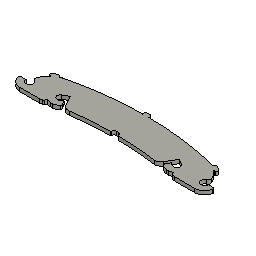
top-piece (Autodesk Fusion 360 design; units mm, degrees)
Autodesk Fusion 360 part; units mm, degrees
note: some values were not read from the file. Set by a fixed rule: which sketch regions a step uses.
(part 1 of 2)
sketch "Main body" plane through (0, 0, 0) normal (0, 0, 1) x (1, 0, 0)
  line L0 (0, 0) -> (0, 30.7494) construction
  line L1 (60, 23.4426) -> (-60, 23.4426) construction
  line L2 (-70, 13.4426) -> (70, 13.4426) construction
  line L3 (-70, 13.4426) -> (-70, 0) construction
  line L4 (70, 0) -> (70, 13.4426) construction
  line L5 (-77.5, 7.9426) -> (77.5, 7.9426) construction
  circle A0 centre (-70, 7.9426) radius 2.9426 construction
  arc A1 (-77.8598, 6.7985) -> (-70, 0) centre (-70, 7.9426) ccw
  line L6 (-76.8702, 7.9426) -> (-72.9426, 7.9426)
  arc A2 (-76.8702, 7.9426) -> (-77.8598, 6.7985) centre (-76.8702, 6.9426) ccw
  circle A3 centre (70, 7.9426) radius 2.9426 construction
  line L7 (72.9426, 7.9426) -> (76.8702, 7.9426)
  arc A4 (70, 0) -> (77.8598, 6.7985) centre (70, 7.9426) ccw
  arc A5 (77.8598, 6.7985) -> (76.8702, 7.9426) centre (76.8702, 6.9426) ccw
  arc A6 (-72.9426, 7.9426) -> (-68.8487, 10.6506) centre (-70, 7.9426) ccw
  arc A7 (68.8487, 10.6506) -> (72.9426, 7.9426) centre (70, 7.9426) ccw
  line L8 (-77.5, 30.7494) -> (77.5, 30.7494) construction
  line L9 (77.5, 30.7494) -> (77.5, 0) construction
  line L10 (77.5, 0) -> (-77.5, 0) construction
  line L11 (-77.5, 0) -> (-77.5, 30.7494) construction
  line L12 (-60, 23.4426) -> (-60, 13.4426) construction
  line L13 (60, 23.4426) -> (60, 13.4426) construction
  line L14 (-70, 0) -> (70, 0)
  arc A8 (59.6571, 23.5271) -> (-59.6571, 23.5271) centre (0, -219.2506) ccw
  arc A9 (-60.3719, 23.2864) -> (-70, 13.4426) centre (-53.134, 6.5765) ccw
  arc A10 (-70, 13.4426) -> (-68.8487, 10.6506) centre (-68.0067, 12.6311) ccw
  line L15 (-60, 13.4426) -> (-66.0104, 19.453) construction
  arc A11 (70, 13.4426) -> (60.3719, 23.2864) centre (53.134, 6.5765) ccw
  line L16 (66.0105, 19.4529) -> (60, 13.4426) construction
  arc A12 (68.8487, 10.6506) -> (70, 13.4426) centre (68.0067, 12.6311) ccw
  arc A13 (-59.6571, 23.5271) -> (-60.3719, 23.2864) centre (-58.5833, 19.1571) ccw
  arc A14 (60.3719, 23.2864) -> (59.6571, 23.5271) centre (58.5833, 19.1571) ccw
  point P0 (0, 13.4426)
  point P1 (0, 7.9426)
  point P2 (70, 7.9426)
  point P3 (-72.9426, 7.9426)
  point P4 (72.9426, 7.9426)
  point P5 (-77.5, 7.9426)
  point P6 (-77.5, 13.4426)
  point P7 (-77.5, 23.4426)
  point P8 (-70, 0)
  point P9 (0, 30.7494)
  point P10 (-70, 30.7494)
  point P11 (-60, 30.7494)
  point P12 (0, 30.2837)
  point P13 (-66.6872, 16.948)
  point P14 (-66.0104, 19.453)
  dimension "d450" = 5.8852
  dimension "d456" = 1
  dimension "d457" = 5.8852
  dimension "d458" = 1
  dimension "d459" = 7.9426
  dimension "d460" = 5.5
  dimension "d461" = 10
  dimension "d463" = 70
  dimension "d465" = 7.5
  dimension "d467" = 10
  dimension "d520" = 250
  dimension "d551" = 8.5
  dimension "d552" = 8.5
  dimension "d561" = 4.5
  dimension "d562" = 4.5
  dimension "d572" = 2.1521
  dimension "d573" = 2.1521
  dimension "d574" = 10
  constraint coincident L0.start origin
  constraint vertical L0
  constraint perpendicular L0 L1
  constraint horizontal L2
  constraint coincident L2 P0
  constraint midpoint L2 P0
  constraint coincident L0 P0
  constraint perpendicular L2 L3
  constraint perpendicular L4 L5
  constraint coincident L5 P1
  constraint midpoint L5 P1
  constraint coincident L0 P1
  constraint coincident L5 A0.centre
  constraint coincident L3 A0.centre
  constraint coincident L5 P2
  constraint coincident L4 P2
  constraint coincident A0.centre A1.centre
  constraint coincident L5 L6.start
  constraint coincident L5 P3
  constraint parallel L5 L6
  constraint coincident A0 P3
  constraint coincident P3 L6.end
  constraint coincident A1.start A2.end
  constraint tangent L6 A2
  constraint tangent A1 A2
  constraint coincident P2 A3.centre
  constraint coincident L5 P4
  constraint coincident L5 L7.end
  constraint parallel L5 L7
  constraint coincident A3 P4
  constraint coincident P4 L7.start
  constraint tangent L5 A5
  constraint tangent A4 A5
  constraint coincident A0 A6.end
  constraint horizontal L8
  constraint vertical L9
  constraint horizontal L10
  constraint vertical L11
  constraint coincident L11 P5
  constraint coincident L11 P6
  constraint coincident L11 P7
  constraint coincident L10 P8
  constraint midpoint L0.start L10
  constraint coincident L5 P5
  constraint coincident L2 P6
  constraint coincident L1 P7
  constraint midpoint L8 P9
  constraint coincident L8 P10
  constraint coincident L3 P10
  constraint coincident P5 L5.start
  constraint coincident L3 P8
  constraint coincident P9 L0.end
  constraint coincident L2 L12.end
  constraint perpendicular L2 L12
  constraint coincident L2 L13.end
  constraint perpendicular L2 L13
  constraint coincident L8 P11
  constraint coincident L12 P11
  constraint coincident A1 P8
  constraint coincident L4.start L10
  constraint coincident P8 L3.end
  constraint perpendicular L0 L5
  constraint coincident L0 P12
  constraint tangent A9 A10
  constraint tangent A0 A10
  constraint coincident P14 L15.end
  constraint tangent A11 A12
  constraint tangent A7 A12
  constraint coincident P9 A8
  constraint coincident A9 P14
  constraint coincident L1.end A8
  constraint coincident L1.end A9
  constraint tangent A8 A13
  constraint tangent A9 A13
  constraint coincident A11 L16.start
  constraint coincident L1.start A8
  constraint coincident L1.start A11
  constraint tangent A8 A14
  constraint tangent A11 A14
  measures "d450" diameter of A0
  measures "d456" radius of A2
  measures "d457" diameter of A3
  measures "d458" radius of A5
  measures "d459" distance of L10.end P5
  measures "d460" distance of P5 P6
  measures "d461" distance of P6 P7
  measures "d463" distance of P9 P10
  measures "d465" distance of L8.start P10
  measures "d467" distance of P10 P11
  measures "d520" radius of A8
  measures "d551" distance of L12.end P14
  measures "d552" distance of L13.end L16.start
  measures "d561" radius of A13
  measures "d562" radius of A14
  measures "d572" radius of A12
  measures "d573" radius of A10
  measures "d574" distance of L2.end L13.end
sketch "Inner connectors _ old" plane through (0, 0, 0) normal (0, 0, 1) x (1, 0, 0)
  line L0 (-77.5, 7.9426) -> (77.5, 7.9426) construction
  line L1 (77.5, 0) -> (-77.5, 0) construction
  line L2 (-77.5, 0) -> (77.5, 0) construction
  line L3 (-35.4314, 0) -> (-43.4022, 13.8057)
  line L4 (-37.9718, 0) -> (-42.5574, 7.9426) construction
  line L5 (-43.5574, 7.9426) -> (-42.5574, 7.9426) construction
  line L6 (-40.6522, 9.0426) -> (-42.5574, 7.9426) construction
  arc A0 (-45.5, 5.1751) -> (-43.5574, 7.9426) centre (-46.5, 7.9426) ccw
  arc A1 (-46.5, 0) -> (-40.3845, 2.8745) centre (-46.5, 7.9426) ccw
  line L7 (-46.5, 7.9426) -> (-46.5, 0) construction
  arc A2 (-40.3845, 2.8745) -> (-40.2884, 4.0126) centre (-41.1545, 3.5126) ccw
  line L8 (-46.5, 0) -> (-35.4314, 0)
  line L9 (35.6624, 0) -> (43.5754, 13.7057)
  line L10 (37.9718, 0) -> (42.5574, 7.9426) construction
  line L11 (43.5574, 7.9426) -> (42.5574, 7.9426) construction
  line L12 (42.5574, 7.9426) -> (40.8254, 8.9426) construction
  arc A3 (43.5574, 7.9426) -> (45.5, 5.1751) centre (46.5, 7.9426) ccw
  arc A4 (40.3845, 2.8745) -> (46.5, 0) centre (46.5, 7.9426) ccw
  arc A5 (40.2884, 4.0126) -> (40.3845, 2.8745) centre (41.1545, 3.5126) ccw
  line L13 (46.5, 7.9426) -> (46.5, 0) construction
  line L14 (35.6624, 0) -> (46.5, 0)
  line L15 (-47.5, 5.1751) -> (-45.5, 5.1751)
  line L16 (-40.2884, 4.0126) -> (-42.0574, 7.0766)
  arc A6 (-42.0574, 7.0766) -> (-43.5574, 7.9426) centre (-43.5574, 6.2105) ccw
  line L17 (40.2884, 4.0126) -> (42.0574, 7.0766)
  arc A7 (43.5574, 7.9426) -> (42.0574, 7.0766) centre (43.5574, 6.2105) ccw
  line L18 (47.5, 5.1751) -> (45.5, 5.1751)
  line L19 (43.5754, 13.7057) -> (47.3852, 11.5061)
  arc A8 (-49.4426, 7.9426) -> (-47.5, 5.1751) centre (-46.5, 7.9426) ccw
  line L20 (-43.4022, 13.8057) -> (-47.3852, 11.5061)
  arc A9 (-47.3852, 11.5061) -> (-49.4426, 7.9426) centre (-45.3277, 7.9426) ccw
  arc A10 (47.5, 5.1751) -> (49.4426, 7.9426) centre (46.5, 7.9426) ccw
  arc A11 (49.4426, 7.9426) -> (47.3852, 11.5061) centre (45.3277, 7.9426) ccw
  point P0 (-70, 7.9426)
  point P1 (70, 7.9426)
  point P2 (-46.5, 5.1751)
  point P3 (46.5, 5.1751)
  point P4 (-43.4022, 13.8057)
  dimension "d469" = 23.5
  dimension "d471" = 23.5
  dimension "d486" = 60
  dimension "d487" = 2.2
  dimension "d488" = 1
  dimension "d492" = 1
  dimension "d493" = 60
  dimension "d495" = 1
  dimension "d498" = 2
  dimension "d500" = 1
  dimension "d571" = 5
  dimension "d575" = 2.9426
  dimension "d577" = 1
  dimension "d578" = 1
  dimension "d579" = 2.9426
  dimension "d585" = 5
  constraint coincident L1.end L2.start
  constraint coincident L1.start L2.end
  constraint coincident L1 L3.start
  constraint coincident L1 L4.start
  constraint parallel L3 L4
  constraint coincident L0 L5.start
  constraint parallel L0 L5
  constraint coincident L3 L6.start
  constraint perpendicular L3 L6
  constraint coincident L2 A1.start
  constraint coincident A0.centre A1.centre
  constraint vertical L7
  constraint tangent A1 A2
  constraint coincident L4 A2.end
  constraint coincident L2 L9.start
  constraint coincident L2 L10.start
  constraint parallel L9 L10
  constraint coincident L0 L11.start
  constraint parallel L0 L11
  constraint perpendicular L10 L12
  constraint coincident L9 L12.end
  constraint coincident L2 A4.end
  constraint coincident A3.centre A4.centre
  constraint coincident L10 A5.start
  constraint tangent L10 A5
  constraint tangent A4 A5
  constraint coincident L1 A4.end
  constraint perpendicular L1 L13
  constraint coincident A0 L15.end
  constraint horizontal L15
  constraint coincident L4 L16.end
  constraint tangent A2 L16
  constraint parallel L4 L16
  constraint tangent L16 A6
  constraint coincident L10 L17.end
  constraint parallel L10 L17
  constraint tangent L17 A7
  constraint tangent L0 A6
  constraint tangent L0 A7
  constraint coincident A3 L18.end
  constraint horizontal L18
  constraint perpendicular L9 L19
  constraint coincident A0.start L15.end
  constraint coincident L0 A0.centre
  constraint midpoint L15 P2
  constraint coincident L7 P2
  constraint coincident L0 A3.centre
  constraint midpoint L18 P3
  constraint coincident L13 P3
  constraint coincident A3.end L18.end
  constraint coincident P4 L3.end
  constraint coincident L0 A8.start
  constraint coincident A8.start A9.end
  constraint coincident L20.end A9.start
  constraint tangent A8 A9
  constraint tangent L20 A9
  constraint perpendicular L3 L20
  constraint tangent A10 A11
  constraint tangent L19 A11
  constraint coincident L0 A10.end
  measures "d469" distance of P0 A0.centre
  measures "d471" distance of P1 A3.centre
  measures "d486" angle of L2 L3
  measures "d487" distance of L3 L4
  measures "d488" distance of L5.start L4.end
  measures "d492" radius of A2
  measures "d493" angle of L2 L10
  measures "d495" distance of L11.start L10.end
  measures "d498" distance of L10.end L12.end
  measures "d500" radius of A5
  measures "d571" distance of L11.start L19
  measures "d575" radius of A0
  measures "d577" distance of L15.start P2
  measures "d578" distance of L13 A3.end
  measures "d579" radius of A3
  measures "d585" distance of L5.start L20
sketch "Inner curve" plane through (0, 0, 0) normal (0, 0, 1) x (1, 0, 0)
  line L0 (-70, 0) -> (70, 0) construction
  line L1 (0, 30.7494) -> (0, 0) construction
  arc A0 (59.6571, 23.5271) -> (-59.6571, 23.5271) centre (0, -219.2506) ccw
  arc A1 (53.3069, 0) -> (-53.3069, 0) centre (0, -244.2506) ccw
  line L2 (-70, 0) -> (70, 0) construction
  line L3 (-53.3069, 0) -> (53.3069, 0)
  point P0 (0, 30.7494)
  point P1 (0, 5.7494)
  dimension "d505" = 25
  dimension "d586" = 250
  constraint coincident P0 L1.start
  constraint coincident L1.end origin
  constraint coincident L1 P1
  constraint coincident L0 A1.start
  constraint coincident L0 A1.end
  constraint midpoint P1 A1
  constraint coincident L0.start L2.start
  constraint coincident L0.end L2.end
  measures "d505" distance of P0 P1
  measures "d586" radius of A1
sketch "Spike top" plane through (0, 0, 0) normal (0, 0, 1) x (1, 0, 0)
  arc A0 (-1, 33.2494) -> (-2.5, 31.7494) centre (-1, 31.7494) ccw
  line L0 (2.5, 31.7494) -> (2.5, 30.7369)
  line L1 (-1, 33.2494) -> (1, 33.2494)
  arc A1 (2.5, 31.7494) -> (1, 33.2494) centre (1, 31.7494) ccw
  line L2 (-2.5, 30.7369) -> (-2.5, 31.7494)
  line L3 (0, 0) -> (0, 33.2494) construction
  arc A2 (59.6571, 23.5271) -> (-59.6571, 23.5271) centre (0, -219.2506) ccw
  point P0 (2.5, 33.2494)
  point P1 (-2.5, 33.2494)
  point P2 (0, 30.7494)
  dimension "d196" = 5
  dimension "d198" = 1.5
  dimension "d199" = 1.5
  dimension "d522" = 2.5
  constraint vertical L2
  constraint perpendicular L1 L2
  constraint vertical L0
  constraint coincident P1 L2
  constraint coincident P1 L1
  constraint tangent A0 L2
  constraint tangent A0 L1
  constraint coincident P0 L1
  constraint coincident P0 L0
  constraint tangent L1 A1
  constraint tangent L0 A1
  constraint coincident L3.start origin
  constraint vertical L3
  constraint midpoint L1 L3.end
  constraint coincident L2.start A2
  constraint coincident L0.end A2
  constraint coincident P2 A2
  measures "d196" distance of P0 P1
  measures "d198" radius of A0
  measures "d199" radius of A1
  measures "d522" distance of L3.end P2
sketch "Spike side" plane through (0, 0, 0) normal (0, 0, 1) x (1, 0, 0)
  line L0 (-64.6665, 23.7784) -> (-63.2744, 21.7019) construction
  line L1 (-66.8617, 22.3068) -> (-62.4714, 25.2501) construction
  line L2 (-66.8617, 22.3068) -> (-68.0588, 21.5042) construction
  line L3 (-62.4714, 25.2501) -> (-61.2782, 22.8639) construction
  line L4 (-68.0588, 21.5042) -> (-66.0092, 19.4542) construction
  arc A0 (-61.4625, 23.2324) -> (-64.3452, 23.9939) centre (-63.2391, 22.344) ccw
  arc A1 (-66.5432, 22.5203) -> (-66.7687, 20.2138) centre (-65.7079, 21.2744) ccw
  line L5 (-66.5432, 22.5203) -> (-64.3452, 23.9939)
  line L6 (-61.4625, 23.2324) -> (-61.2782, 22.8639)
  line L7 (-66.4461, 19.8912) -> (-61.4625, 23.2324) construction
  line L8 (-65.6155, 20.4481) -> (-65.3622, 20.0701)
  line L9 (-65.6155, 20.4481) -> (-66.4461, 19.8912)
  line L10 (-66.7687, 20.2138) -> (-66.4461, 19.8912)
  line L11 (66.8617, 22.3068) -> (62.4714, 25.2501) construction
  line L12 (66.4461, 19.8912) -> (61.4625, 23.2324) construction
  line L13 (66.8617, 22.3068) -> (68.0588, 21.5042) construction
  line L14 (64.6665, 23.7784) -> (63.2744, 21.7019) construction
  line L15 (62.4714, 25.2501) -> (61.2782, 22.8639) construction
  line L16 (65.6155, 20.4481) -> (66.4461, 19.8912)
  arc A2 (66.5432, 22.5203) -> (66.7687, 20.2138) centre (65.7079, 21.2744) cw
  line L17 (66.5432, 22.5203) -> (64.3452, 23.9939)
  line L18 (65.6155, 20.4481) -> (65.3622, 20.0701)
  arc A3 (61.4625, 23.2324) -> (64.3452, 23.9939) centre (63.2391, 22.344) cw
  line L19 (61.4625, 23.2324) -> (61.2782, 22.8639)
  line L20 (68.0588, 21.5042) -> (66.0092, 19.4542) construction
  line L21 (66.7687, 20.2138) -> (66.4461, 19.8912)
  arc A4 (-60.3719, 23.2864) -> (-70, 13.4426) centre (-53.134, 6.5765) ccw
  arc A5 (70, 13.4426) -> (60.3719, 23.2864) centre (53.134, 6.5765) ccw
  point P0 (0, 47.6931)
  point P1 (0, 45.6174)
  point P2 (-53.134, 6.5765)
  point P3 (-66.0104, 19.453)
  point P4 (53.134, 6.5765)
  point P5 (66.0105, 19.4529)
  dimension "d314" = 2.5
  dimension "d321" = 1.5
  dimension "d323" = 2.5
  dimension "d327" = 1.5
  dimension "d553" = 0.455
  dimension "d554" = 0.455
  dimension "d555" = 5
  dimension "d556" = 1
  dimension "d557" = 5
  dimension "d558" = 1
  dimension "d559" = 1
  dimension "d560" = 1
  constraint midpoint L0.start L1
  constraint perpendicular L0 L1
  constraint collinear L1 L2
  constraint tangent L1 A0
  constraint coincident L3 A0.start
  constraint coincident L1 A0.end
  constraint tangent L3 A0
  constraint coincident L4 A1.end
  constraint coincident L1 A1.start
  constraint tangent L1 A1
  constraint tangent L4 A1
  constraint coincident L4 L7.start
  constraint coincident L7 L8.start
  constraint perpendicular L7 L8
  constraint coincident L1.start L8
  constraint midpoint L14.start L11
  constraint perpendicular L11 L14
  constraint collinear L11 L13
  constraint tangent L11 A3
  constraint coincident L12.end L15
  constraint coincident L17.end L11
  constraint tangent L15 A3
  constraint coincident A2.end L20
  constraint coincident A2.start L11
  constraint tangent L11 A2
  constraint tangent A2 L20
  constraint coincident L12.start L20
  constraint coincident L16.start L12
  constraint perpendicular L12 L18
  constraint coincident L11.start L18
  constraint perpendicular L0 L7
  constraint coincident L12.end L19
  constraint perpendicular L12 L14
  constraint coincident L3.end A4
  constraint coincident L0.end A4
  constraint coincident L4.end A4
  constraint coincident L0 P2
  constraint coincident L14 P4
  constraint coincident L18.end A5
  constraint coincident L20.end A5
  constraint coincident L14.end A5
  constraint coincident L15 P4
  constraint coincident L20 P4
  constraint coincident L4 P2
  constraint coincident L3 P2
  constraint coincident L8.end A4
  constraint coincident A5 L15.end
  measures "d314" distance of L0.start L0.end
  measures "d321" radius of A1
  measures "d323" distance of L14.end L14.start
  measures "d327" radius of A2
  measures "d553" distance of L8.start L8.end
  measures "d554" distance of L18.end L16.start
  measures "d555" distance of A0.start L8.start
  measures "d556" distance of L7.start L8.start
  measures "d557" distance of L12.end L16.start
  measures "d558" distance of L12.start L16.start
  measures "d559" distance of L3.end A4.start
  measures "d560" distance of A5.end L15.end
sketch "Inner connector" plane through (0, 0, 0) normal (0, 0, 1) x (1, 0, 0)
  arc A0 (53.3069, 0) -> (-53.3069, 0) centre (0, -244.2506) ccw
  line L0 (-70, 7.9426) -> (-46.5, 7.9426) construction
  line L1 (-46.5, 9.4539) -> (-46.5, 1.3868) construction
  arc A1 (-45.5, 6.6865) -> (-43.9516, 7.9827) centre (-46.5, 9.4539) ccw
  line L2 (-45.5, 6.6865) -> (-47.5, 6.6865)
  arc A2 (-49.0248, 7.9426) -> (-47.5, 6.6865) centre (-46.5, 9.4539) ccw
  line L3 (-39.0403, 5.876) -> (-43.6804, 13.9128)
  line L4 (-46.5, 9.4539) -> (-51.7672, 0.331) construction
  line L5 (-43.6804, 13.9128) -> (-48.1443, 11.3355)
  line L6 (-46.5, 9.4539) -> (-43.9516, 7.9827) construction
  line L7 (-43.9516, 7.9827) -> (-43.0856, 8.4827)
  line L8 (-45.5, 6.6865) -> (-45.5, 1.6865) construction
  line L9 (-47.5, 6.6865) -> (-47.5, 1.6865) construction
  line L10 (-47.5, 1.6865) -> (-45.5, 1.6865)
  arc A3 (-45.5, 1.6865) -> (-41.2154, 3.6741) centre (-46.5, 9.4539) ccw
  arc A4 (-50.4158, 2.6716) -> (-47.5, 1.6865) centre (-46.5, 9.4539) ccw
  line L11 (-50.4158, 2.6716) -> (-51.4694, 0.8467)
  arc A5 (-48.1443, 11.3355) -> (-49.0248, 7.9426) centre (-46.9147, 9.2057) ccw
  line L12 (-43.0856, 8.4827) -> (-41.0242, 4.9121)
  arc A6 (-41.2154, 3.6741) -> (-41.0242, 4.9121) centre (-41.8902, 4.4121) ccw
  arc A7 (-39.0403, 5.876) -> (-34.0296, 3.4225) centre (-34.7102, 8.376) ccw
  line L13 (0, 0) -> (0, 5.7494)
  arc A8 (47.5, 1.6865) -> (50.4158, 2.6716) centre (46.5, 9.4539) ccw
  line L14 (47.5, 1.6865) -> (45.5, 1.6865)
  arc A9 (41.2154, 3.6741) -> (45.5, 1.6865) centre (46.5, 9.4539) ccw
  arc A10 (41.0242, 4.9121) -> (41.2154, 3.6741) centre (41.8902, 4.4121) ccw
  line L15 (43.0856, 8.4827) -> (41.0242, 4.9121)
  line L16 (43.9516, 7.9827) -> (43.0856, 8.4827)
  arc A11 (43.9516, 7.9827) -> (45.5, 6.6865) centre (46.5, 9.4539) ccw
  line L17 (45.5, 6.6865) -> (47.5, 6.6865)
  arc A12 (47.5, 6.6865) -> (49.0248, 7.9426) centre (46.5, 9.4539) ccw
  arc A13 (49.0248, 7.9426) -> (48.1443, 11.3355) centre (46.9147, 9.2057) ccw
  line L18 (43.6804, 13.9128) -> (48.1443, 11.3355)
  line L19 (39.0403, 5.876) -> (43.6804, 13.9128)
  arc A14 (34.0296, 3.4225) -> (39.0403, 5.876) centre (34.7102, 8.376) ccw
  line L20 (-45.5, 1.6865) -> (-45.5, 1.574) construction
  line L21 (77.5, 0) -> (-77.5, 0) construction
  line L22 (-51.7672, 0.331) -> (-53.3069, 0) construction
  arc A15 (-52.1253, 0.3691) -> (-51.4694, 0.8467) centre (-52.3354, 1.3467) ccw
  line L23 (-53.8422, 0) -> (-52.1253, 0.3691)
  line L24 (-53.3069, 0) -> (-53.8422, 0)
  line L25 (50.4158, 2.6716) -> (51.4694, 0.8467)
  arc A16 (51.4694, 0.8467) -> (52.1253, 0.3691) centre (52.3354, 1.3467) ccw
  line L26 (53.8422, 0) -> (52.1253, 0.3691)
  line L27 (53.3069, 0) -> (53.8422, 0)
  point P0 (-70, 7.9426)
  point P1 (-46.5, 6.6865)
  point P2 (-45.5, 6.6865)
  dimension "d598" = 23.5
  dimension "d617" = 2.9426
  dimension "d618" = 2
  dimension "d620" = 1
  dimension "d623" = 30
  dimension "d624" = 5
  dimension "d625" = 60
  dimension "d633" = 30
  dimension "d634" = 2.2
  dimension "d635" = 1
  dimension "d637" = 5
  dimension "d639" = 23.5
  dimension "d658" = 0.1125
  dimension "d662" = 1
  dimension "d663" = 5
  dimension "d664" = 0.1125
  constraint coincident P0 L0.start
  constraint coincident L0.end L1
  constraint coincident A0 L1.end
  constraint vertical L1
  constraint horizontal L0
  constraint coincident L1 A1.centre
  constraint perpendicular L1 L2
  constraint midpoint L2 P1
  constraint coincident L1 P1
  constraint coincident P2 A1.start
  constraint coincident L1.start A1.centre
  constraint coincident A0 L4.end
  constraint perpendicular L3 L5
  constraint perpendicular L2 L8
  constraint perpendicular L2 L9
  constraint horizontal L10
  constraint parallel L4 L11
  constraint tangent L5 A5
  constraint tangent A2 A5
  constraint coincident L0 A2.start
  constraint perpendicular L7 L12
  constraint parallel L3 L12
  constraint tangent L12 A6
  constraint tangent A3 A6
  constraint tangent L3 A7
  constraint coincident A0 A7.end
  constraint tangent A0 A7
  constraint coincident L13.start origin
  constraint midpoint A0 L13.end
  constraint symmetric P2 L13 A11.end
  constraint symmetric A1.end L13 L16.start
  constraint symmetric A1 L13 A11
  constraint symmetric L2.end L13 L17.end
  constraint symmetric A2.start L13 A12.end
  constraint symmetric A2 L13 A12
  constraint symmetric L3.start L13 L19.start
  constraint symmetric L3.end L13 L18.start
  constraint symmetric L5.end L13 A13.end
  constraint symmetric L7.end L13 L15.start
  constraint symmetric L8.end L13 L14.end
  constraint symmetric L9.end L13 A8.start
  constraint symmetric A3.end L13 A9.start
  constraint symmetric A3 L13 A9
  constraint symmetric A4.start L13 A8.end
  constraint symmetric A4 L13 A8
  constraint symmetric A5 L13 A13
  constraint symmetric L12.end L13 A10.start
  constraint symmetric A6 L13 A10
  constraint symmetric A7.end L13 A14.start
  constraint symmetric A7 L13 A14
  constraint coincident A0 L20.end
  constraint perpendicular L10 L20
  constraint coincident L8.end L10.end
  constraint coincident A0.end L22.end
  constraint coincident L21 L23.start
  constraint tangent L4 A15
  constraint coincident L4 L11.end
  constraint coincident L11 A15.end
  constraint parallel L22 L23
  constraint parallel L21 L24
  constraint coincident L11.end A15.end
  constraint tangent A15 L23
  constraint symmetric L13 A0.end A0.start
  constraint symmetric L13 L23.start L26.start
  constraint symmetric L13 L11.end L25.end
  constraint symmetric L13 A15.start A16.end
  constraint symmetric L13 A15 A16
  measures "d598" distance of P0 L0.end
  measures "d617" radius of A1
  measures "d618" distance of P2 L2.end
  measures "d620" distance of A1.end L7.end
  measures "d623" angle of L1 L4
  measures "d624" distance of A1.end L5
  measures "d625" angle of L1 L6
  measures "d633" angle of L1 L3
  measures "d634" distance of L3 L7.end
  measures "d635" radius of A6
  measures "d637" radius of A7
  measures "d639" distance of P0 L0.end
  measures "d658" distance of L8.end L20.end
  measures "d662" radius of A15
  measures "d663" distance of P2 L8.end
  measures "d664" distance of L22 L23
extrude "Extrude6" add sketch "Spike top" sketch "Main body" sketch "Spike side" along normal blind 3 of sketch 2 of sketch 3 makes body 1
extrude "Extrude7" cut sketch "Inner connector" sketch "Inner curve" along normal blind 3 of sketch 2 bodies 1
copy_body "CopyPasteBodies6" bodies 1 makes body 2
move_body "Move9" bodies 2 to x (1, 0, 0) y (0, 1, 0) z (0, 0, 1) at (0, -25.45, 0)
sketch "Cutouts" plane through (0, 0, 0) normal (0, 0, 1) x (1, 0, 0)
  line L0 (-70, 0) -> (70, 0)
  arc A0 (-1, 7.7994) -> (-2.5, 6.2994) centre (-1, 6.2994) ccw construction
  line L1 (-2.5, 6.2994) -> (-2.5, 5.2869) construction
  line L2 (1, 7.7994) -> (-1, 7.7994) construction
  arc A1 (2.5, 6.2994) -> (1, 7.7994) centre (1, 6.2994) ccw construction
  line L3 (2.5, 5.2869) -> (2.5, 6.2994) construction
  line L4 (2.95, 5.2869) -> (2.95, 6.2994)
  arc A2 (2.95, 6.2994) -> (1, 8.2494) centre (1, 6.2994) ccw
  line L5 (1, 8.2494) -> (-1, 8.2494)
  arc A3 (-1, 8.2494) -> (-2.95, 6.2994) centre (-1, 6.2994) ccw
  line L6 (-2.95, 6.2994) -> (-2.95, 5.2869)
  line L7 (-2.95, 5.2869) -> (-2.95, 0)
  line L8 (2.95, 5.2869) -> (2.95, 0)
  dimension "d527" = 0.45
  constraint coincident L0 L7.end
  constraint perpendicular L0 L7
  constraint coincident L0 L8.end
  constraint perpendicular L0 L8
extrude "Extrude8" cut sketch "Cutouts" along normal blind 3 bodies 1
delete_body "RemoveBody3" bodies 2
sketch "Without inner connectors" plane through (0, 0, 0) normal (0, 0, 1) x (1, 0, 0)
  line L0 (2.95, 6.2994) -> (2.95, 5.732)
  line L1 (53.3069, 0) -> (70, 0)
  arc A0 (70, 0) -> (77.8598, 6.7985) centre (70, 7.9426) ccw
  arc A1 (77.8598, 6.7985) -> (76.8702, 7.9426) centre (76.8702, 6.9426) ccw
  line L2 (76.8702, 7.9426) -> (72.9426, 7.9426)
  arc A2 (68.8487, 10.6506) -> (72.9426, 7.9426) centre (70, 7.9426) ccw
  arc A3 (68.8487, 10.6506) -> (70, 13.4426) centre (68.0067, 12.6311) ccw
  arc A4 (70, 13.4426) -> (65.3622, 20.0701) centre (53.134, 6.5765) ccw
  line L3 (65.3622, 20.0701) -> (65.6155, 20.4481)
  line L4 (65.6155, 20.4481) -> (66.4461, 19.8912)
  line L5 (66.4461, 19.8912) -> (66.7687, 20.2138)
  arc A5 (66.7687, 20.2138) -> (66.5432, 22.5203) centre (65.7079, 21.2744) ccw
  line L6 (66.5432, 22.5203) -> (64.3452, 23.9939)
  arc A6 (64.3452, 23.9939) -> (61.4625, 23.2324) centre (63.2391, 22.344) ccw
  line L7 (61.4625, 23.2324) -> (61.2782, 22.8639)
  arc A7 (61.2782, 22.8639) -> (60.3719, 23.2864) centre (53.134, 6.5765) ccw
  arc A8 (60.3719, 23.2864) -> (59.6571, 23.5271) centre (58.5833, 19.1571) ccw
  arc A9 (59.6571, 23.5271) -> (2.5, 30.7369) centre (0, -219.2506) ccw
  line L8 (2.5, 30.7369) -> (2.5, 31.7494)
  arc A10 (2.5, 31.7494) -> (1, 33.2494) centre (1, 31.7494) ccw
  line L9 (1, 33.2494) -> (-1, 33.2494)
  arc A11 (-1, 33.2494) -> (-2.5, 31.7494) centre (-1, 31.7494) ccw
  line L10 (-2.5, 31.7494) -> (-2.5, 30.7369)
  arc A12 (-2.5, 30.7369) -> (-59.6571, 23.5271) centre (0, -219.2506) ccw
  arc A13 (-59.6571, 23.5271) -> (-60.3719, 23.2864) centre (-58.5833, 19.1571) ccw
  arc A14 (-60.3719, 23.2864) -> (-61.2782, 22.8639) centre (-53.134, 6.5765) ccw
  line L11 (-61.2782, 22.8639) -> (-61.4625, 23.2324)
  arc A15 (-61.4625, 23.2324) -> (-64.3452, 23.9939) centre (-63.2391, 22.344) ccw
  line L12 (-64.3452, 23.9939) -> (-66.5432, 22.5203)
  arc A16 (-66.5432, 22.5203) -> (-66.7687, 20.2138) centre (-65.7079, 21.2744) ccw
  line L13 (-66.7687, 20.2138) -> (-66.4461, 19.8912)
  line L14 (-66.4461, 19.8912) -> (-65.6155, 20.4481)
  line L15 (-65.6155, 20.4481) -> (-65.3622, 20.0701)
  arc A17 (-65.3622, 20.0701) -> (-70, 13.4426) centre (-53.134, 6.5765) ccw
  arc A18 (-70, 13.4426) -> (-68.8487, 10.6506) centre (-68.0067, 12.6311) ccw
  arc A19 (-72.9426, 7.9426) -> (-68.8487, 10.6506) centre (-70, 7.9426) ccw
  line L16 (-72.9426, 7.9426) -> (-76.8702, 7.9426)
  arc A20 (-76.8702, 7.9426) -> (-77.8598, 6.7985) centre (-76.8702, 6.9426) ccw
  arc A21 (-77.8598, 6.7985) -> (-70, 0) centre (-70, 7.9426) ccw
  line L17 (-70, 0) -> (-53.3069, 0)
  line L18 (-2.95, 5.732) -> (-2.95, 6.2994)
  arc A22 (-1, 8.2494) -> (-2.95, 6.2994) centre (-1, 6.2994) ccw
  line L19 (-1, 8.2494) -> (1, 8.2494)
  arc A23 (2.95, 6.2994) -> (1, 8.2494) centre (1, 6.2994) ccw
  arc A24 (41.3805, 2.3009) -> (36.4767, 3.0739) centre (0, -244.2506) ccw
  arc A25 (-36.4767, 3.0739) -> (-41.0722, 2.3524) centre (0, -244.2506) ccw
  arc A26 (53.3069, 0) -> (2.95, 5.732) centre (0, -244.2506) ccw
  arc A27 (-2.95, 5.732) -> (-53.3069, 0) centre (0, -244.2506) ccw
  dimension "d592" = 250
  dimension "d593" = 250
  measures "d592" radius of A24
  measures "d593" radius of A25
sketch "Inner connectors isolated" plane through (0, 0, 0) normal (0, 0, 1) x (1, 0, 0)
  arc A0 (-36.4767, 3.0739) -> (-41.0722, 2.3524) centre (0, -244.2506) ccw
  arc A1 (41.3805, 2.3009) -> (36.4767, 3.0739) centre (0, -244.2506) ccw
  arc A2 (53.3069, 0) -> (2.95, 5.732) centre (0, -244.2506) ccw
  arc A3 (-2.95, 5.732) -> (-53.3069, 0) centre (0, -244.2506) ccw
  dimension "d594" = 250
  dimension "d595" = 250
  measures "d594" radius of A0
  measures "d595" radius of A1
copy_body "Body->Comp3" bodies 1 removing the originals makes body 3 in component "Component"
sketch "Kerf offsets" plane through (0, 0, 0) normal (0, 0, 1) x (1, 0, 0)
  line L0 (2.95, 31.7494) -> (2.95, 31.182)
  arc A0 (34.0296, 28.8725) -> (2.95, 31.182) centre (0, -218.8006) ccw
  arc A1 (34.0296, 28.8725) -> (39.0403, 31.326) centre (34.7102, 33.826) ccw
  line L1 (39.0403, 31.326) -> (43.6804, 39.3628)
  line L2 (43.6804, 39.3628) -> (48.1443, 36.7855)
  arc A2 (49.0248, 33.3926) -> (48.1443, 36.7855) centre (46.9147, 34.6557) ccw
  arc A3 (47.5, 32.1365) -> (49.0248, 33.3926) centre (46.5, 34.9039) ccw
  line L3 (47.5, 32.1365) -> (45.5, 32.1365)
  arc A4 (43.9516, 33.4327) -> (45.5, 32.1365) centre (46.5, 34.9039) ccw
  line L4 (43.9516, 33.4327) -> (43.0856, 33.9327)
  line L5 (43.0856, 33.9327) -> (41.0242, 30.3621)
  arc A5 (41.0242, 30.3621) -> (41.2154, 29.1241) centre (41.8902, 29.8621) ccw
  arc A6 (41.2154, 29.1241) -> (45.5, 27.1365) centre (46.5, 34.9039) ccw
  line L6 (45.5, 27.1365) -> (47.5, 27.1365)
  arc A7 (47.5, 27.1365) -> (50.4158, 28.1216) centre (46.5, 34.9039) ccw
  line L7 (50.4158, 28.1216) -> (51.4694, 26.2967)
  arc A8 (51.4694, 26.2967) -> (52.1253, 25.8191) centre (52.3354, 26.7967) ccw
  line L8 (52.1253, 25.8191) -> (53.8422, 25.45)
  line L9 (53.8422, 25.45) -> (70, 25.45)
  arc A9 (70, 25.45) -> (77.8598, 32.2485) centre (70, 33.3926) ccw
  arc A10 (77.8598, 32.2485) -> (76.8702, 33.3926) centre (76.8702, 32.3926) ccw
  line L10 (76.8702, 33.3926) -> (72.9426, 33.3926)
  arc A11 (68.8487, 36.1006) -> (72.9426, 33.3926) centre (70, 33.3926) ccw
  arc A12 (68.8487, 36.1006) -> (70, 38.8926) centre (68.0067, 38.0811) ccw
  arc A13 (70, 38.8926) -> (65.3622, 45.5201) centre (53.134, 32.0265) ccw
  line L11 (65.3622, 45.5201) -> (65.6155, 45.8981)
  line L12 (65.6155, 45.8981) -> (66.4461, 45.3412)
  line L13 (66.4461, 45.3412) -> (66.7687, 45.6638)
  arc A14 (66.7687, 45.6638) -> (66.5432, 47.9703) centre (65.7079, 46.7244) ccw
  line L14 (66.5432, 47.9703) -> (64.3452, 49.4439)
  arc A15 (64.3452, 49.4439) -> (61.4625, 48.6824) centre (63.2391, 47.794) ccw
  line L15 (61.4625, 48.6824) -> (61.2782, 48.3139)
  arc A16 (61.2782, 48.3139) -> (60.3719, 48.7364) centre (53.134, 32.0265) ccw
  arc A17 (60.3719, 48.7364) -> (59.6571, 48.9771) centre (58.5833, 44.6071) ccw
  arc A18 (59.6571, 48.9771) -> (2.5, 56.1869) centre (0, -193.8006) ccw
  line L16 (2.5, 56.1869) -> (2.5, 57.1994)
  arc A19 (2.5, 57.1994) -> (1, 58.6994) centre (1, 57.1994) ccw
  line L17 (1, 58.6994) -> (-1, 58.6994)
  arc A20 (-1, 58.6994) -> (-2.5, 57.1994) centre (-1, 57.1994) ccw
  line L18 (-2.5, 57.1994) -> (-2.5, 56.1869)
  arc A21 (-2.5, 56.1869) -> (-59.6571, 48.9771) centre (0, -193.8006) ccw
  arc A22 (-59.6571, 48.9771) -> (-60.3719, 48.7364) centre (-58.5833, 44.6071) ccw
  arc A23 (-60.3719, 48.7364) -> (-61.2782, 48.3139) centre (-53.134, 32.0265) ccw
  line L19 (-61.2782, 48.3139) -> (-61.4625, 48.6824)
  arc A24 (-61.4625, 48.6824) -> (-64.3452, 49.4439) centre (-63.2391, 47.794) ccw
  line L20 (-64.3452, 49.4439) -> (-66.5432, 47.9703)
  arc A25 (-66.5432, 47.9703) -> (-66.7687, 45.6638) centre (-65.7079, 46.7244) ccw
  line L21 (-66.7687, 45.6638) -> (-66.4461, 45.3412)
  line L22 (-66.4461, 45.3412) -> (-65.6155, 45.8981)
  line L23 (-65.6155, 45.8981) -> (-65.3622, 45.5201)
  arc A26 (-65.3622, 45.5201) -> (-70, 38.8926) centre (-53.134, 32.0265) ccw
  arc A27 (-70, 38.8926) -> (-68.8487, 36.1006) centre (-68.0067, 38.0811) ccw
  arc A28 (-72.9426, 33.3926) -> (-68.8487, 36.1006) centre (-70, 33.3926) ccw
  line L24 (-72.9426, 33.3926) -> (-76.8702, 33.3926)
  arc A29 (-76.8702, 33.3926) -> (-77.8598, 32.2485) centre (-76.8702, 32.3926) ccw
  arc A30 (-77.8598, 32.2485) -> (-70, 25.45) centre (-70, 33.3926) ccw
  line L25 (-70, 25.45) -> (-53.8422, 25.45)
  line L26 (-53.8422, 25.45) -> (-52.1253, 25.8191)
  arc A31 (-52.1253, 25.8191) -> (-51.4694, 26.2967) centre (-52.3354, 26.7967) ccw
  line L27 (-51.4694, 26.2967) -> (-50.4158, 28.1216)
  arc A32 (-50.4158, 28.1216) -> (-47.5, 27.1365) centre (-46.5, 34.9039) ccw
  line L28 (-47.5, 27.1365) -> (-45.5, 27.1365)
  arc A33 (-45.5, 27.1365) -> (-41.2154, 29.1241) centre (-46.5, 34.9039) ccw
  arc A34 (-41.2154, 29.1241) -> (-41.0242, 30.3621) centre (-41.8902, 29.8621) ccw
  line L29 (-41.0242, 30.3621) -> (-43.0856, 33.9327)
  line L30 (-43.0856, 33.9327) -> (-43.9516, 33.4327)
  arc A35 (-45.5, 32.1365) -> (-43.9516, 33.4327) centre (-46.5, 34.9039) ccw
  line L31 (-45.5, 32.1365) -> (-47.5, 32.1365)
  arc A36 (-49.0248, 33.3926) -> (-47.5, 32.1365) centre (-46.5, 34.9039) ccw
  arc A37 (-48.1443, 36.7855) -> (-49.0248, 33.3926) centre (-46.9147, 34.6557) ccw
  line L32 (-48.1443, 36.7855) -> (-43.6804, 39.3628)
  line L33 (-43.6804, 39.3628) -> (-39.0403, 31.326)
  arc A38 (-39.0403, 31.326) -> (-34.0296, 28.8725) centre (-34.7102, 33.826) ccw
  arc A39 (-2.95, 31.182) -> (-34.0296, 28.8725) centre (0, -218.8006) ccw
  line L34 (-2.95, 31.182) -> (-2.95, 31.7494)
  arc A40 (-1, 33.6994) -> (-2.95, 31.7494) centre (-1, 31.7494) ccw
  line L35 (-1, 33.6994) -> (1, 33.6994)
  arc A41 (2.95, 31.7494) -> (1, 33.6994) centre (1, 31.7494) ccw
  line L36 (2.95, 6.2994) -> (2.95, 5.732)
  arc A42 (34.0296, 3.4225) -> (2.95, 5.732) centre (0, -244.2506) ccw
  arc A43 (34.0296, 3.4225) -> (39.0403, 5.876) centre (34.7102, 8.376) ccw
  line L37 (39.0403, 5.876) -> (43.6804, 13.9128)
  line L38 (43.6804, 13.9128) -> (48.1443, 11.3355)
  arc A44 (49.0248, 7.9426) -> (48.1443, 11.3355) centre (46.9147, 9.2057) ccw
  arc A45 (47.5, 6.6865) -> (49.0248, 7.9426) centre (46.5, 9.4539) ccw
  line L39 (47.5, 6.6865) -> (45.5, 6.6865)
  arc A46 (43.9516, 7.9827) -> (45.5, 6.6865) centre (46.5, 9.4539) ccw
  line L40 (43.9516, 7.9827) -> (43.0856, 8.4827)
  line L41 (43.0856, 8.4827) -> (41.0242, 4.9121)
  arc A47 (41.0242, 4.9121) -> (41.2154, 3.6741) centre (41.8902, 4.4121) ccw
  arc A48 (41.2154, 3.6741) -> (45.5, 1.6865) centre (46.5, 9.4539) ccw
  line L42 (45.5, 1.6865) -> (47.5, 1.6865)
  arc A49 (47.5, 1.6865) -> (50.4158, 2.6716) centre (46.5, 9.4539) ccw
  line L43 (50.4158, 2.6716) -> (51.4694, 0.8467)
  arc A50 (51.4694, 0.8467) -> (52.1253, 0.3691) centre (52.3354, 1.3467) ccw
  line L44 (52.1253, 0.3691) -> (53.8422, 0)
  line L45 (53.8422, 0) -> (70, 0)
  arc A51 (70, 0) -> (77.8598, 6.7985) centre (70, 7.9426) ccw
  arc A52 (77.8598, 6.7985) -> (76.8702, 7.9426) centre (76.8702, 6.9426) ccw
  line L46 (76.8702, 7.9426) -> (72.9426, 7.9426)
  arc A53 (68.8487, 10.6506) -> (72.9426, 7.9426) centre (70, 7.9426) ccw
  arc A54 (68.8487, 10.6506) -> (70, 13.4426) centre (68.0067, 12.6311) ccw
  arc A55 (70, 13.4426) -> (65.3622, 20.0701) centre (53.134, 6.5765) ccw
  line L47 (65.3622, 20.0701) -> (65.6155, 20.4481)
  line L48 (65.6155, 20.4481) -> (66.4461, 19.8912)
  line L49 (66.4461, 19.8912) -> (66.7687, 20.2138)
  arc A56 (66.7687, 20.2138) -> (66.5432, 22.5203) centre (65.7079, 21.2744) ccw
  line L50 (66.5432, 22.5203) -> (64.3452, 23.9939)
  arc A57 (64.3452, 23.9939) -> (61.4625, 23.2324) centre (63.2391, 22.344) ccw
  line L51 (61.4625, 23.2324) -> (61.2782, 22.8639)
  arc A58 (61.2782, 22.8639) -> (60.3719, 23.2864) centre (53.134, 6.5765) ccw
  arc A59 (60.3719, 23.2864) -> (59.6571, 23.5271) centre (58.5833, 19.1571) ccw
  arc A60 (59.6571, 23.5271) -> (2.5, 30.7369) centre (0, -219.2506) ccw
  line L52 (2.5, 30.7369) -> (2.5, 31.7494)
  arc A61 (2.5, 31.7494) -> (1, 33.2494) centre (1, 31.7494) ccw
  line L53 (1, 33.2494) -> (-1, 33.2494)
  arc A62 (-1, 33.2494) -> (-2.5, 31.7494) centre (-1, 31.7494) ccw
  line L54 (-2.5, 31.7494) -> (-2.5, 30.7369)
  arc A63 (-2.5, 30.7369) -> (-59.6571, 23.5271) centre (0, -219.2506) ccw
  arc A64 (-59.6571, 23.5271) -> (-60.3719, 23.2864) centre (-58.5833, 19.1571) ccw
  arc A65 (-60.3719, 23.2864) -> (-61.2782, 22.8639) centre (-53.134, 6.5765) ccw
  line L55 (-61.2782, 22.8639) -> (-61.4625, 23.2324)
  arc A66 (-61.4625, 23.2324) -> (-64.3452, 23.9939) centre (-63.2391, 22.344) ccw
  line L56 (-64.3452, 23.9939) -> (-66.5432, 22.5203)
  arc A67 (-66.5432, 22.5203) -> (-66.7687, 20.2138) centre (-65.7079, 21.2744) ccw
  line L57 (-66.7687, 20.2138) -> (-66.4461, 19.8912)
  line L58 (-66.4461, 19.8912) -> (-65.6155, 20.4481)
  line L59 (-65.6155, 20.4481) -> (-65.3622, 20.0701)
  arc A68 (-65.3622, 20.0701) -> (-70, 13.4426) centre (-53.134, 6.5765) ccw
  arc A69 (-70, 13.4426) -> (-68.8487, 10.6506) centre (-68.0067, 12.6311) ccw
  arc A70 (-72.9426, 7.9426) -> (-68.8487, 10.6506) centre (-70, 7.9426) ccw
  line L60 (-72.9426, 7.9426) -> (-76.8702, 7.9426)
  arc A71 (-76.8702, 7.9426) -> (-77.8598, 6.7985) centre (-76.8702, 6.9426) ccw
  arc A72 (-77.8598, 6.7985) -> (-70, 0) centre (-70, 7.9426) ccw
  line L61 (-70, 0) -> (-53.8422, 0)
  line L62 (-53.8422, 0) -> (-52.1253, 0.3691)
  arc A73 (-52.1253, 0.3691) -> (-51.4694, 0.8467) centre (-52.3354, 1.3467) ccw
  line L63 (-51.4694, 0.8467) -> (-50.4158, 2.6716)
  arc A74 (-50.4158, 2.6716) -> (-47.5, 1.6865) centre (-46.5, 9.4539) ccw
  line L64 (-47.5, 1.6865) -> (-45.5, 1.6865)
  arc A75 (-45.5, 1.6865) -> (-41.2154, 3.6741) centre (-46.5, 9.4539) ccw
  arc A76 (-41.2154, 3.6741) -> (-41.0242, 4.9121) centre (-41.8902, 4.4121) ccw
  line L65 (-41.0242, 4.9121) -> (-43.0856, 8.4827)
  line L66 (-43.0856, 8.4827) -> (-43.9516, 7.9827)
  arc A77 (-45.5, 6.6865) -> (-43.9516, 7.9827) centre (-46.5, 9.4539) ccw
  line L67 (-45.5, 6.6865) -> (-47.5, 6.6865)
  arc A78 (-49.0248, 7.9426) -> (-47.5, 6.6865) centre (-46.5, 9.4539) ccw
  arc A79 (-48.1443, 11.3355) -> (-49.0248, 7.9426) centre (-46.9147, 9.2057) ccw
  line L68 (-48.1443, 11.3355) -> (-43.6804, 13.9128)
  line L69 (-43.6804, 13.9128) -> (-39.0403, 5.876)
  arc A80 (-39.0403, 5.876) -> (-34.0296, 3.4225) centre (-34.7102, 8.376) ccw
  arc A81 (-2.95, 5.732) -> (-34.0296, 3.4225) centre (0, -244.2506) ccw
  line L70 (-2.95, 5.732) -> (-2.95, 6.2994)
  arc A82 (-1, 8.2494) -> (-2.95, 6.2994) centre (-1, 6.2994) ccw
  line L71 (-1, 8.2494) -> (1, 8.2494)
  arc A83 (2.95, 6.2994) -> (1, 8.2494) centre (1, 6.2994) ccw
  arc A84 (-50.3319, 27.817) -> (-47.5143, 26.9115) centre (-46.5, 34.9039) ccw
  line L72 (-47.5143, 26.9115) -> (-45.4857, 26.9115)
  arc A85 (-45.4857, 26.9115) -> (-41.0636, 28.9581) centre (-46.5, 34.9039) ccw
  arc A86 (-41.0636, 28.9581) -> (-40.8293, 30.4746) centre (-41.8902, 29.8621) ccw
  line L73 (-40.8293, 30.4746) -> (-43.0033, 34.24)
  line L74 (-43.0033, 34.24) -> (-44.1175, 33.5967)
  arc A87 (-45.5402, 32.3615) -> (-44.1175, 33.5967) centre (-46.5, 34.9039) ccw
  line L75 (-45.5402, 32.3615) -> (-47.4598, 32.3615)
  arc A88 (-48.8317, 33.5081) -> (-47.4598, 32.3615) centre (-46.5, 34.9039) ccw
  arc A89 (-48.0318, 36.5907) -> (-48.8317, 33.5081) centre (-46.9147, 34.6557) ccw
  line L76 (-48.0318, 36.5907) -> (-43.7627, 39.0554)
  line L77 (-43.7627, 39.0554) -> (-39.2352, 31.2135)
  arc A90 (-39.2352, 31.2135) -> (-33.999, 28.6496) centre (-34.7102, 33.826) ccw
  arc A91 (-2.725, 30.9595) -> (-33.999, 28.6496) centre (0, -218.8006) ccw
  line L78 (-2.725, 30.9595) -> (-2.725, 31.7494)
  arc A92 (-1, 33.4744) -> (-2.725, 31.7494) centre (-1, 31.7494) ccw
  line L79 (-1, 33.4744) -> (1, 33.4744)
  arc A93 (2.725, 31.7494) -> (1, 33.4744) centre (1, 31.7494) ccw
  line L80 (2.725, 31.7494) -> (2.725, 30.9595)
  arc A94 (33.999, 28.6496) -> (2.725, 30.9595) centre (0, -218.8006) ccw
  arc A95 (33.999, 28.6496) -> (39.2352, 31.2135) centre (34.7102, 33.826) ccw
  line L81 (39.2352, 31.2135) -> (43.7627, 39.0554)
  line L82 (43.7627, 39.0554) -> (48.0318, 36.5907)
  arc A96 (48.8317, 33.5081) -> (48.0318, 36.5907) centre (46.9147, 34.6557) ccw
  arc A97 (47.4598, 32.3615) -> (48.8317, 33.5081) centre (46.5, 34.9039) ccw
  line L83 (47.4598, 32.3615) -> (45.5402, 32.3615)
  arc A98 (44.1175, 33.5967) -> (45.5402, 32.3615) centre (46.5, 34.9039) ccw
  line L84 (44.1175, 33.5967) -> (43.0033, 34.24)
  line L85 (43.0033, 34.24) -> (40.8293, 30.4746)
  arc A99 (40.8293, 30.4746) -> (41.0636, 28.9581) centre (41.8902, 29.8621) ccw
  arc A100 (41.0636, 28.9581) -> (45.4857, 26.9115) centre (46.5, 34.9039) ccw
  line L86 (45.4857, 26.9115) -> (47.5143, 26.9115)
  arc A101 (47.5143, 26.9115) -> (50.3319, 27.817) centre (46.5, 34.9039) ccw
  line L87 (50.3319, 27.817) -> (51.2745, 26.1842)
  arc A102 (51.2745, 26.1842) -> (52.078, 25.5991) centre (52.3354, 26.7967) ccw
  line L88 (52.078, 25.5991) -> (53.8183, 25.225)
  line L89 (53.8183, 25.225) -> (70, 25.225)
  arc A103 (70, 25.225) -> (78.0824, 32.2161) centre (70, 33.3926) ccw
  arc A104 (78.0824, 32.2161) -> (76.8702, 33.6176) centre (76.8702, 32.3926) ccw
  line L90 (76.8702, 33.6176) -> (72.7083, 33.6176)
  arc A105 (68.9368, 35.8935) -> (72.7083, 33.6176) centre (70, 33.3926) ccw
  arc A106 (68.9368, 35.8935) -> (70.2084, 38.9774) centre (68.0067, 38.0811) ccw
  arc A107 (70.2084, 38.9774) -> (65.6567, 45.5555) centre (53.134, 32.0265) ccw
  line L91 (65.6567, 45.5555) -> (65.6771, 45.5859)
  line L92 (65.6771, 45.5859) -> (66.4745, 45.0513)
  line L93 (66.4745, 45.0513) -> (66.9278, 45.5047)
  arc A108 (66.9278, 45.5047) -> (66.6685, 48.1572) centre (65.7079, 46.7244) ccw
  line L94 (66.6685, 48.1572) -> (64.4705, 49.6307)
  arc A109 (64.4705, 49.6307) -> (61.2612, 48.783) centre (63.2391, 47.794) ccw
  line L95 (61.2612, 48.783) -> (61.177, 48.6145)
  arc A110 (61.177, 48.6145) -> (60.4613, 48.9428) centre (53.134, 32.0265) ccw
  arc A111 (60.4613, 48.9428) -> (59.7108, 49.1956) centre (58.5833, 44.6071) ccw
  arc A112 (59.7108, 49.1956) -> (2.725, 56.4095) centre (0, -193.8006) ccw
  line L96 (2.725, 56.4095) -> (2.725, 57.1994)
  arc A113 (2.725, 57.1994) -> (1, 58.9244) centre (1, 57.1994) ccw
  line L97 (1, 58.9244) -> (-1, 58.9244)
  arc A114 (-1, 58.9244) -> (-2.725, 57.1994) centre (-1, 57.1994) ccw
  line L98 (-2.725, 57.1994) -> (-2.725, 56.4095)
  arc A115 (-2.725, 56.4095) -> (-59.7108, 49.1956) centre (0, -193.8006) ccw
  arc A116 (-59.7108, 49.1956) -> (-60.4613, 48.9428) centre (-58.5833, 44.6071) ccw
  arc A117 (-60.4613, 48.9428) -> (-61.177, 48.6145) centre (-53.134, 32.0265) ccw
  line L99 (-61.177, 48.6145) -> (-61.2612, 48.783)
  arc A118 (-61.2612, 48.783) -> (-64.4705, 49.6307) centre (-63.2391, 47.794) ccw
  line L100 (-64.4705, 49.6307) -> (-66.6685, 48.1572)
  arc A119 (-66.6685, 48.1572) -> (-66.9278, 45.5047) centre (-65.7079, 46.7244) ccw
  line L101 (-66.9278, 45.5047) -> (-66.4745, 45.0513)
  line L102 (-66.4745, 45.0513) -> (-65.6771, 45.5859)
  line L103 (-65.6771, 45.5859) -> (-65.6567, 45.5555)
  arc A120 (-65.6567, 45.5555) -> (-70.2084, 38.9774) centre (-53.134, 32.0265) ccw
  arc A121 (-70.2084, 38.9774) -> (-68.9368, 35.8935) centre (-68.0067, 38.0811) ccw
  arc A122 (-72.7083, 33.6176) -> (-68.9368, 35.8935) centre (-70, 33.3926) ccw
  line L104 (-72.7083, 33.6176) -> (-76.8702, 33.6176)
  arc A123 (-76.8702, 33.6176) -> (-78.0824, 32.2161) centre (-76.8702, 32.3926) ccw
  arc A124 (-78.0824, 32.2161) -> (-70, 25.225) centre (-70, 33.3926) ccw
  line L105 (-70, 25.225) -> (-53.8183, 25.225)
  line L106 (-53.8183, 25.225) -> (-52.078, 25.5991)
  arc A125 (-52.078, 25.5991) -> (-51.2745, 26.1842) centre (-52.3354, 26.7967) ccw
  line L107 (-51.2745, 26.1842) -> (-50.3319, 27.817)
  arc A126 (-50.3319, 2.367) -> (-47.5143, 1.4615) centre (-46.5, 9.4539) ccw
  line L108 (-47.5143, 1.4615) -> (-45.4857, 1.4615)
  arc A127 (-45.4857, 1.4615) -> (-41.0636, 3.5081) centre (-46.5, 9.4539) ccw
  arc A128 (-41.0636, 3.5081) -> (-40.8293, 5.0246) centre (-41.8902, 4.4121) ccw
  line L109 (-40.8293, 5.0246) -> (-43.0033, 8.79)
  line L110 (-43.0033, 8.79) -> (-44.1175, 8.1467)
  arc A129 (-45.5402, 6.9115) -> (-44.1175, 8.1467) centre (-46.5, 9.4539) ccw
  line L111 (-45.5402, 6.9115) -> (-47.4598, 6.9115)
  arc A130 (-48.8317, 8.0581) -> (-47.4598, 6.9115) centre (-46.5, 9.4539) ccw
  arc A131 (-48.0318, 11.1407) -> (-48.8317, 8.0581) centre (-46.9147, 9.2057) ccw
  line L112 (-48.0318, 11.1407) -> (-43.7627, 13.6054)
  line L113 (-43.7627, 13.6054) -> (-39.2352, 5.7635)
  arc A132 (-39.2352, 5.7635) -> (-33.999, 3.1996) centre (-34.7102, 8.376) ccw
  arc A133 (-2.725, 5.5095) -> (-33.999, 3.1996) centre (0, -244.2506) ccw
  line L114 (-2.725, 5.5095) -> (-2.725, 6.2994)
  arc A134 (-1, 8.0244) -> (-2.725, 6.2994) centre (-1, 6.2994) ccw
  line L115 (-1, 8.0244) -> (1, 8.0244)
  arc A135 (2.725, 6.2994) -> (1, 8.0244) centre (1, 6.2994) ccw
  line L116 (2.725, 6.2994) -> (2.725, 5.5095)
  arc A136 (33.999, 3.1996) -> (2.725, 5.5095) centre (0, -244.2506) ccw
  arc A137 (33.999, 3.1996) -> (39.2352, 5.7635) centre (34.7102, 8.376) ccw
  line L117 (39.2352, 5.7635) -> (43.7627, 13.6054)
  line L118 (43.7627, 13.6054) -> (48.0318, 11.1407)
  arc A138 (48.8317, 8.0581) -> (48.0318, 11.1407) centre (46.9147, 9.2057) ccw
  arc A139 (47.4598, 6.9115) -> (48.8317, 8.0581) centre (46.5, 9.4539) ccw
  line L119 (47.4598, 6.9115) -> (45.5402, 6.9115)
  arc A140 (44.1175, 8.1467) -> (45.5402, 6.9115) centre (46.5, 9.4539) ccw
  line L120 (44.1175, 8.1467) -> (43.0033, 8.79)
  line L121 (43.0033, 8.79) -> (40.8293, 5.0246)
  arc A141 (40.8293, 5.0246) -> (41.0636, 3.5081) centre (41.8902, 4.4121) ccw
  arc A142 (41.0636, 3.5081) -> (45.4857, 1.4615) centre (46.5, 9.4539) ccw
  line L122 (45.4857, 1.4615) -> (47.5143, 1.4615)
  arc A143 (47.5143, 1.4615) -> (50.3319, 2.367) centre (46.5, 9.4539) ccw
  line L123 (50.3319, 2.367) -> (51.2745, 0.7342)
  arc A144 (51.2745, 0.7342) -> (52.078, 0.1491) centre (52.3354, 1.3467) ccw
  line L124 (52.078, 0.1491) -> (53.8183, -0.225)
  line L125 (53.8183, -0.225) -> (70, -0.225)
  arc A145 (70, -0.225) -> (78.0824, 6.7661) centre (70, 7.9426) ccw
  arc A146 (78.0824, 6.7661) -> (76.8702, 8.1676) centre (76.8702, 6.9426) ccw
  line L126 (76.8702, 8.1676) -> (72.7083, 8.1676)
  arc A147 (68.9368, 10.4435) -> (72.7083, 8.1676) centre (70, 7.9426) ccw
  arc A148 (68.9368, 10.4435) -> (70.2084, 13.5274) centre (68.0067, 12.6311) ccw
  arc A149 (70.2084, 13.5274) -> (65.6567, 20.1055) centre (53.134, 6.5765) ccw
  line L127 (65.6567, 20.1055) -> (65.6771, 20.1359)
  line L128 (65.6771, 20.1359) -> (66.4745, 19.6013)
  line L129 (66.4745, 19.6013) -> (66.9278, 20.0547)
  arc A150 (66.9278, 20.0547) -> (66.6685, 22.7072) centre (65.7079, 21.2744) ccw
  line L130 (66.6685, 22.7072) -> (64.4705, 24.1807)
  arc A151 (64.4705, 24.1807) -> (61.2612, 23.333) centre (63.2391, 22.344) ccw
  line L131 (61.2612, 23.333) -> (61.177, 23.1645)
  arc A152 (61.177, 23.1645) -> (60.4613, 23.4928) centre (53.134, 6.5765) ccw
  arc A153 (60.4613, 23.4928) -> (59.7108, 23.7456) centre (58.5833, 19.1571) ccw
  arc A154 (59.7108, 23.7456) -> (2.725, 30.9595) centre (0, -219.2506) ccw
  line L132 (2.725, 30.9595) -> (2.725, 31.7494)
  arc A155 (2.725, 31.7494) -> (1, 33.4744) centre (1, 31.7494) ccw
  line L133 (1, 33.4744) -> (-1, 33.4744)
  arc A156 (-1, 33.4744) -> (-2.725, 31.7494) centre (-1, 31.7494) ccw
  line L134 (-2.725, 31.7494) -> (-2.725, 30.9595)
  arc A157 (-2.725, 30.9595) -> (-59.7108, 23.7456) centre (0, -219.2506) ccw
  arc A158 (-59.7108, 23.7456) -> (-60.4613, 23.4928) centre (-58.5833, 19.1571) ccw
  arc A159 (-60.4613, 23.4928) -> (-61.177, 23.1645) centre (-53.134, 6.5765) ccw
  line L135 (-61.177, 23.1645) -> (-61.2612, 23.333)
  arc A160 (-61.2612, 23.333) -> (-64.4705, 24.1807) centre (-63.2391, 22.344) ccw
  line L136 (-64.4705, 24.1807) -> (-66.6685, 22.7072)
  arc A161 (-66.6685, 22.7072) -> (-66.9278, 20.0547) centre (-65.7079, 21.2744) ccw
  line L137 (-66.9278, 20.0547) -> (-66.4745, 19.6013)
  line L138 (-66.4745, 19.6013) -> (-65.6771, 20.1359)
  line L139 (-65.6771, 20.1359) -> (-65.6567, 20.1055)
  arc A162 (-65.6567, 20.1055) -> (-70.2084, 13.5274) centre (-53.134, 6.5765) ccw
  arc A163 (-70.2084, 13.5274) -> (-68.9368, 10.4435) centre (-68.0067, 12.6311) ccw
  arc A164 (-72.7083, 8.1676) -> (-68.9368, 10.4435) centre (-70, 7.9426) ccw
  line L140 (-72.7083, 8.1676) -> (-76.8702, 8.1676)
  arc A165 (-76.8702, 8.1676) -> (-78.0824, 6.7661) centre (-76.8702, 6.9426) ccw
  arc A166 (-78.0824, 6.7661) -> (-70, -0.225) centre (-70, 7.9426) ccw
  line L141 (-70, -0.225) -> (-53.8183, -0.225)
  line L142 (-53.8183, -0.225) -> (-52.078, 0.1491)
  arc A167 (-52.078, 0.1491) -> (-51.2745, 0.7342) centre (-52.3354, 1.3467) ccw
  line L143 (-51.2745, 0.7342) -> (-50.3319, 2.367)
  dimension "d665" = 0.225
  dimension "d666" = 0.225